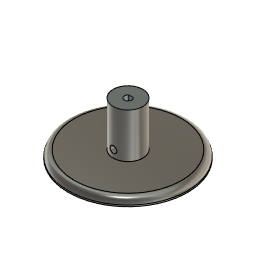
Spool Final (Autodesk Fusion 360 design; units mm, degrees)
Autodesk Fusion 360 part; units mm, degrees
sketch "Sketch1" plane through (0, 0, 0) normal (0, 0, 1) x (1, 0, 0)
  line L0 (1.5, 2) -> (-1.5, 2)
  arc A0 (-1.5, 2) -> (1.5, 2) centre (0, 0) ccw
cylinder "CylinderPrimitive1" add diameter 80 height 5 placed x (1, 0, 0) y (0, 1, 0) z (0, 0, 1) at (0, 0, 0) makes body 1
cylinder "CylinderPrimitive2" add diameter 20 height 30 placed x (1, 0, 0) y (0, 1, 0) z (0, 0, 1) at (0, 0, 5) bodies 1
extrude "Extrude1" cut sketch "Sketch1" along normal blind 44 bodies 1
fillet "Fillet1" radius 4 1 edges at (-37.2931, -14.4646, 5) on bodies 1
sketch "Sketch4" plane through (0, 0, 35) normal (0, 0, 1) x (-1, 0, 0)
  line L0 (1.5, -2) -> (-1.5, -2)
  arc A0 (1.5, -2) -> (-1.5, -2) centre (0, 0) ccw
  circle A1 centre (0, 0) radius 10
cylinder "CylinderPrimitive3" add diameter 4.5 height 31 placed x (1, 0, 0) y (0, 0, -1) z (0, 1, 0) at (0, 0, 10) separate body makes body 2
move_body "Move1" bodies 2 to x (1, 0, 0) y (0, 1, 0) z (0, 0, 1) at (0, -16, 0)
combine "Combine1" operation cut target body 1 tool bodies 2
